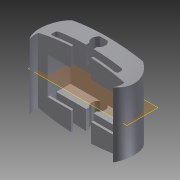
# Autodesk Inventor part: chasis
Saved by Autodesk Inventor 2012 (Build 160160000, 160)
## iProperties
Created: 2012-12-28
Part Number: chasis
Material: Default
Document SubType Name: Modeling
Designer: otrebor
Density: 1 g/cm^3
Author: otrebor
Autodesk Inventor part; units mm, degrees
ref_plane "YZ Plane" through (0, 0, 0) normal (1, 0, 0) x (0, 1, 0)
ref_plane "XZ Plane" through (0, 0, 0) normal (0, 1, 0) x (-1, 0, 0)
ref_plane "XY Plane" through (0, 0, 0) normal (0, 0, 1) x (1, 0, 0)
sketch "Boceto1" plane through (0, 0, 0) normal (0, 0, 1) x (1, 0, 0)
  line L0 (-3.4214, 5.0502) -> (3.4219, 5.0498)
  arc A0 (-3.4214, 5.0502) -> (-3.4219, -5.0498) centre (0, 0) ccw
  arc A1 (3.4214, -5.0502) -> (3.4219, 5.0498) centre (0, 0) ccw
  line L1 (56.2152, -10.9474) -> (-53.9546, -10.9418) construction
  line L2 (0.0842, 24.332) -> (0.0818, -24.0148) construction
  arc A2 (-32.9166, 8.05) -> (-38.4881, -25.2963) centre (-21.8149, -10.9435) ccw
  arc A3 (38.6514, -25.3002) -> (33.0834, 8.0467) centre (21.9797, -10.9457) ccw
  line L3 (4.2598, -8.0502) -> (31.0826, -8.0516)
  line L4 (-3.422, -8.0498) -> (-30.9174, -8.0484)
  line L5 (-8.9764, -14.0495) -> (-30.9177, -14.0484)
  line L6 (-8.9764, -14.0495) -> (-8.9765, -16.0495)
  line L7 (-8.9765, -16.0495) -> (-39.8927, -16.048)
  arc A4 (-39.8927, -16.048) -> (-38.4881, -25.2963) centre (-21.9179, -18.0489) ccw
  line L8 (9.1413, -8.0505) -> (31.0826, -8.0516)
  line L9 (9.141, -14.0505) -> (31.0823, -14.0516)
  line L10 (9.1409, -16.0505) -> (40.057, -16.052)
  line L11 (9.141, -14.0505) -> (9.1409, -16.0505)
  arc A5 (38.6514, -25.3002) -> (40.057, -16.052) centre (22.0821, -18.0511) ccw
  line L12 (-8.9764, -14.0495) -> (-30.9177, -14.0484)
  line L13 (-8.2419, -8.0496) -> (-23.0886, -8.0488) construction
  line L14 (-8.9761, -8.0495) -> (-8.9767, -20.0515) construction
  line L15 (-40.1598, -25.6638) -> (27.0571, -25.6672) construction
  line L16 (27.0571, -25.6672) -> (49.5741, -25.6683) construction
  line L17 (-21.9179, -18.0489) -> (-21.9178, -16.0489) construction
  line L18 (-30.9174, -8.0484) -> (-30.9177, -14.0484)
  line L19 (31.0826, -8.0516) -> (31.0823, -14.0516)
  line L20 (-3.4219, -5.0498) -> (-3.422, -8.0498)
  line L21 (3.4214, -5.0502) -> (3.4212, -8.0502)
  line L22 (-9.0877, -8.0495) -> (-3.422, -8.0498)
  line L23 (3.4212, -8.0502) -> (4.2598, -8.0502)
  line L24 (-32.9166, 8.05) -> (33.0834, 8.0467)
  dimension "d21" = 66
  dimension "d22" = 22
  dimension "d47" = 2
  dimension "d55" = 62
  constraints: 50 end point, 13 point on circle, 10 perpendicular, 9 symmetric about line, 6 centre point, 5 point on line, 2 coincident, 2 collinear, 2 parallel, 2 other
  measures "d21" distance of L24.end L24.start
  measures "d22" radius of A2
  measures "d47" distance of L5.start L6.end
  measures "d55" distance between parallel lines of L19 L18
extrude "Extrusión1" add sketch "Boceto1" along normal blind 70
ref_plane "Plano de trabajo1" through (0, 0, 35) normal (0, 0, 1) x (1, 0, 0)
sketch "Boceto2" plane through (0, 0, 35) normal (0, 0, 1) x (1, 0, 0)
  line L0 (-31.0303, -21.8316) -> (30.9839, -21.8316)
  line L1 (30.9839, -21.8316) -> (30.9839, 5.0579)
  line L2 (30.9839, 5.0579) -> (-31.0303, 5.0579)
  line L3 (-31.0303, 5.0579) -> (-31.0303, -21.8316)
  point P0 (0, 0)
  constraints: 8 end point, 2 parallel, 1 horizontal, 1 perpendicular
extrude "Extrusión2" cut sketch "Boceto2" along normal mid plane 34
fillet "Fillet1" radius 2 1 edges at (-30.9177, -14.0484, 61)
fillet "Fillet2" radius 2 1 edges at (-30.9174, -8.0484, 61)
fillet "Fillet3" radius 2 1 edges at (31.0826, -8.0516, 35)
fillet "Fillet4" radius 2 1 edges at (31.0823, -14.0516, 35)
fillet "Fillet5" radius 1 1 edges at (-8.9764, -14.0495, 61)
fillet "Fillet6" radius 1 1 edges at (9.141, -14.0505, 61)
fillet "Fillet7" radius 1 1 edges at (9.141, -14.0505, 9)
fillet "Fillet8" radius 1 1 edges at (-8.9764, -14.0495, 9)
sketch "Sketch10" plane through (33.0834, 8.0467, 70) normal (0.0000505, 1, 0) x (1, -0.0000505, 0)
  line L0 (-66, 70) -> (-66, 0) projected
  ellipse E0 centre (-33.083, 35) end of major axis (-111.4556, 35) minor radius 34.6629
  line L1 (-66, 0) -> (0, 0) projected
  line L2 (0, 70) -> (0, 0) projected
  line L3 (0, 70) -> (-66, 70) projected
  point P0 (-33.083, 70)
  constraints: 1 vertical, 2 other
extrude "Extrusion9" cut sketch "Sketch10" against normal blind 46.5 contours E0 L2 L0 | L0 E0 | E0 L2 keep common part
sketch "Sketch11" plane through (-32.9166, 8.05, 66.4573) normal (0.0000505, 1, 0) x (1, -0.0000505, 0)
  ellipse E0 centre (32.917, 31.4573) end of major axis (111.2896, 31.4573) minor radius 34.6629 (0, 0) -> (66, 0.0341) ccw projected
  line L0 (66, 62.8806) -> (66, 0.0341) projected
  ellipse E1 centre (32.917, 31.4573) end of major axis (111.2896, 31.4573) minor radius 34.6629 (66, 62.8806) -> (0, 62.9146) ccw projected
  line L1 (0, 62.9146) -> (0, 0) projected
  point P0 (32.917, 66.4573)
  constraints: 2 other
equation "\"d19\" = 0.333333 * d21"
